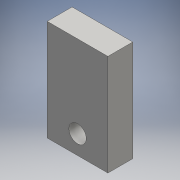
# Autodesk Inventor part: StupidPiece
Saved by Autodesk Inventor 2016 (Build 200138000, 138)
## iProperties
Created: 2017-03-11
Part Number: StupidPiece
Material: Generic
Document SubType Name: Modeling
Designer: Owner
Density: 1 g/cm^3
Appearance: Default
Author: Owner
Autodesk Inventor part; units mm, degrees
ref_plane "YZ Plane" through (0, 0, 0) normal (1, 0, 0) x (0, 1, 0)
ref_plane "XZ Plane" through (0, 0, 0) normal (0, 1, 0) x (-1, 0, 0)
ref_plane "XY Plane" through (0, 0, 0) normal (0, 0, 1) x (1, 0, 0)
sketch "Sketch1" plane through (0, 0, 0) normal (0, 1, 0) x (-1, 0, 0)
  line L0 (12.7, -224.71) -> (0, -224.71)
  line L1 (0, -214.55) -> (12.7, -214.55)
  circle A0 centre (6.35, -220.9) radius 1.75
  circle A1 centre (6.35, -220.9) radius 1.75
  line L2 (12.7, -214.55) -> (12.45, -214.55)
  line L3 (12.45, -214.55) -> (12.45, -224.71)
  line L4 (0, -214.55) -> (0.25, -214.55)
  line L5 (0.25, -214.55) -> (0.25, -224.71)
  point P0 (0, 0)
  dimension "d4" = 0.25
  dimension "d5" = 0.25
  constraints: 12 end point, 4 point on line, 2 centre point, 2 perpendicular, 1 coincident, 1 horizontal, 1 parallel
  measures "d4" distance of L1.end L2.end
  measures "d5" distance of L1.start L4.end
extrude "Extrusion1" add sketch "Sketch1" along normal blind 5.0038
sketch "Sketch2" plane through (-12.7, 0, -214.55) normal (0, 0, 1) x (1, 0, 0)
  line L0 (0.25, 0) -> (12.45, 0) projected
  line L1 (0.25, 5.0038) -> (12.45, 5.0038) projected
  line L2 (12.45, 0) -> (12.45, 5.0038) projected
  line L3 (0.25, 0) -> (0.25, 5.0038) projected
  point P0 (12.7, 0)
extrude "Extrusion2" add sketch "Sketch2" along normal blind 10.16
body "Solid1"
